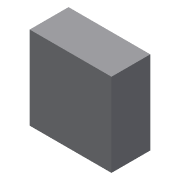
# Autodesk Inventor part: Midsurf - DiffThick
Saved by Autodesk Inventor 2014 (Build 180170000, 170)
## iProperties
Created: 2014-01-16
Part Number: Midsurf - DiffThick
Material: Generic
Document SubType Name: Modeling
Designer: Yogesh
Density: 1 g/cm^3
Appearance: Default
Author: Yogesh
Autodesk Inventor part; units mm, degrees
ref_plane "YZ Plane" through (0, 0, 0) normal (1, 0, 0) x (0, 1, 0)
ref_plane "XZ Plane" through (0, 0, 0) normal (0, 1, 0) x (-1, 0, 0)
ref_plane "XY Plane" through (0, 0, 0) normal (0, 0, 1) x (1, 0, 0)
sketch "Sketch1" plane through (0, 0, 0) normal (0, 1, 0) x (-1, 0, 0)
  line L0 (10.5287, -10.7178) -> (-10.5287, -10.7178)
  line L1 (-10.5287, -10.7178) -> (-10.5287, 10.7178)
  line L2 (-10.5287, 10.7178) -> (10.5287, 10.7178)
  line L3 (10.5287, 10.7178) -> (10.5287, -10.7178)
  line L4 (10.5287, -10.7178) -> (-10.5287, 10.7178) construction
  line L5 (-10.5287, -10.7178) -> (10.5287, 10.7178) construction
  point P0 (0, 0)
  constraints: 12 end point, 2 midpoint, 2 parallel, 1 horizontal, 1 perpendicular
extrude "Extrusion1" add sketch "Sketch1" along normal blind 10
shell "Shell1" thickness 1 removed faces 1 at (-3.5096, 10, -3.5726)
body "Solid1"
